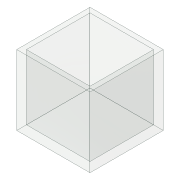
# Autodesk Inventor part: Cuvette_45x45x40
Saved by Autodesk Inventor 2019 (Build 230136000, 136)
## iProperties
Created: 2018-10-04
Part Number: Cuvette_45x45x40
Material: Glass
Document SubType Name: Modeling
Designer: voigt
Density: 2.18 g/cm^3
Appearance: Clear
Author: voigt
Autodesk Inventor part; units mm, degrees
ref_plane "YZ Plane" through (0, 0, 0) normal (1, 0, 0) x (0, 1, 0)
ref_plane "XZ Plane" through (0, 0, 0) normal (0, 1, 0) x (-1, 0, 0)
ref_plane "XY Plane" through (0, 0, 0) normal (0, 0, 1) x (1, 0, 0)
sketch "Sketch1" plane through (0, 0, 0) normal (0, 0, 1) x (1, 0, 0)
  line L0 (0, 31.5) -> (0, -31.5) construction
  line L1 (-31.5, 0) -> (31.5, 0) construction
  line L2 (-19.5, 19.5) -> (19.5, 19.5)
  line L3 (19.5, 19.5) -> (19.5, -19.5)
  line L4 (19.5, -19.5) -> (-19.5, -19.5)
  line L5 (-19.5, -19.5) -> (-19.5, 19.5)
  line L6 (-22.5, 22.5) -> (22.5, 22.5)
  line L7 (22.5, 22.5) -> (22.5, -22.5)
  line L8 (22.5, -22.5) -> (-22.5, -22.5)
  line L9 (-22.5, -22.5) -> (-22.5, 22.5)
  point P0 (0, 0)
  dimension "d0" = 39
  dimension "d1" = 39
  dimension "d2" = 3
  dimension "d3" = 3
  dimension "d4" = 3
  dimension "d5" = 3
  constraints: 16 end point, 4 parallel, 2 horizontal, 2 perpendicular, 2 other
  measures "d0" distance of L2.start L2.end
  measures "d1" distance of L2.end L3.end
  measures "d2" distance between parallel lines of L6 L2
  measures "d3" distance between parallel lines of L5 L9
  measures "d4" distance between parallel lines of L4 L8
  measures "d5" distance between parallel lines of L7 L3
extrude "Extrusion1" add sketch "Sketch1" along normal blind 40
sketch "Sketch2" plane through (0, 0, 0) normal (0, 0, -1) x (-1, 0, 0)
  line L0 (-22.5, -22.5) -> (22.5, -22.5) projected
  line L1 (22.5, -22.5) -> (22.5, 22.5) projected
  line L2 (22.5, 22.5) -> (-22.5, 22.5) projected
  line L3 (-22.5, 22.5) -> (-22.5, -22.5) projected
  point P0 (0, 0)
extrude "Extrusion2" add sketch "Sketch2" along normal blind 3
body "Solid1"
